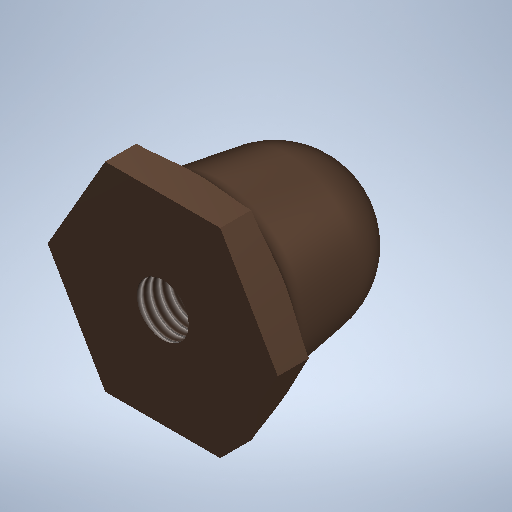
# Autodesk Inventor part: Spinner
Saved by Autodesk Inventor 2025 (Build 290162010, 162A)
## iProperties
Created: 2024-04-30
Part Number: Spinner
Material: Bronze, Cast
Document SubType Name: Modeling
Designer: ffogue
Density: 8.87 g/cm^3
Appearance: Bronze - Satin
Author: ffogue
Autodesk Inventor part; units mm, degrees
ref_plane "YZ Plane" through (0, 0, 0) normal (1, 0, 0) x (0, 1, 0)
ref_plane "XZ Plane" through (0, 0, 0) normal (0, 1, 0) x (-1, 0, 0)
ref_plane "XY Plane" through (0, 0, 0) normal (0, 0, 1) x (1, 0, 0)
sketch "Skizze2" plane through (0, 0, 0) normal (0, 1, 0) x (-1, 0, 0)
  line L0 (18.5, 0) -> (9.25, -16.0215)
  line L1 (9.25, -16.0215) -> (-9.25, -16.0215)
  line L2 (-9.25, -16.0215) -> (-18.5, 0)
  line L3 (-18.5, 0) -> (-9.25, 16.0215)
  line L4 (-9.25, 16.0215) -> (9.25, 16.0215)
  line L5 (9.25, 16.0215) -> (18.5, 0)
  point P0 (0, 0)
  point P1 (0, 0)
  dimension "d8" = 37
  constraints: 12 end point, 1 coincident, 13 other
  measures "d8" distance of L2.end L0.start
extrude "Extrusion1" add sketch "Skizze2" along normal blind 5
sketch "Skizze4" plane through (0, 0, 0) normal (0, 0, 1) x (1, 0, 0)
  line L0 (9.25, 5) -> (-9.25, 5) projected
  line L1 (-9.25, 5) -> (-18.5, 5) projected
  line L2 (18.5, 5) -> (9.25, 5) projected
  arc A0 (-18.5, 5) -> (-13.5631, 9.2083) centre (-18.5, 10) ccw
  line L3 (-13.5631, 9.2083) -> (-11.8486, 19.9)
  arc A1 (0, 30) -> (-11.8486, 19.9) centre (0, 18) ccw
  line L4 (0, 30) -> (0, 0)
  line L5 (9.25, 0) -> (-9.25, 0) projected
  point P0 (0, 5)
  dimension "d11" = 12
  dimension "d12" = 5
  dimension "d13" = 30
  constraints: 4 end point, 4 point on circle, 3 tangent, 2 centre point, 1 point on line, 1 vertical
  measures "d11" radius of A1
  measures "d12" radius of A0
  measures "d13" distance from line of L4.start L5
revolve "Umdrehung1" add sketch "Skizze4" angle 360 about axis through (0, 30, 0) along (0, -1, 0)
sketch "Skizze5" plane through (0, 0, 0) normal (0, -1, 0) x (1, 0, 0)
  line L0 (-9.25, 16.0215) -> (9.25, 16.0215) projected
  line L1 (-18.5, 0) -> (-9.25, 16.0215) projected
  line L2 (-9.25, -16.0215) -> (-18.5, 0) projected
  line L3 (9.25, -16.0215) -> (-9.25, -16.0215) projected
  line L4 (18.5, 0) -> (9.25, -16.0215) projected
  line L5 (9.25, 16.0215) -> (18.5, 0) projected
  arc A0 (-18.5, 0) -> (-9.25, -16.0215) centre (0, 0) ccw projected
  arc A1 (-9.25, 16.0215) -> (-18.5, 0) centre (0, 0) ccw projected
  arc A2 (9.25, 16.0215) -> (-9.25, 16.0215) centre (0, 0) ccw projected
  arc A3 (18.5, 0) -> (9.25, 16.0215) centre (0, 0) ccw projected
  arc A4 (9.25, -16.0215) -> (18.5, 0) centre (0, 0) ccw projected
  line L6 (9.25, -16.0215) -> (-9.25, -16.0215) projected
  arc A5 (-9.25, -16.0215) -> (9.25, -16.0215) centre (0, 0) ccw projected
  point P0 (0, 0)
extrude "Extrusion4" cut sketch "Skizze5" against normal up to surface contours A2 L0 | L1 A1 | A3 L5 | L2 A0 | A4 L4 | L3 A5
sketch "Skizze6" plane through (0, 0, 0) normal (0, -1, 0) x (1, 0, 0)
  point P0 (0, 0)
  point P1 (0, 0)
  constraints: 1 coincident
hole "Bohrung1" at (0, 0, 0) direction (0, 1, 0) diameter 8.376 depth 25 tip angle 118 thread size "M10x1.5" class "6H" standard "ISO Metric profile"
